# Autodesk Inventor part: 7_68MHZ
Saved by Autodesk Inventor 2016 (Build 200138000, 138)
## iProperties
Created: 2016-04-08
Part Number: 7_68MHZ
Material: Generic
Document SubType Name: Modeling
Designer: Paschalis
Density: 1 g/cm^3
Appearance: HC49U-V, 7_68MHZ
Author: Paschalis
Autodesk Inventor part; units mm, degrees
ref_plane "YZ Plane" through (0, 0, 0) normal (1, 0, 0) x (0, 1, 0)
ref_plane "XZ Plane" through (0, 0, 0) normal (0, 1, 0) x (-1, 0, 0)
ref_plane "XY Plane" through (0, 0, 0) normal (0, 0, 1) x (1, 0, 0)
sketch "HC49U-V, 7_68MHZ_85" plane through (0, 0, 0) normal (0, 0, 1) x (1, 0, 0)
  line L0 (-5.588, 2.794) -> (5.588, 2.794)
  line L1 (5.588, 2.794) -> (5.588, -2.794)
  line L2 (5.588, -2.794) -> (-5.588, -2.794)
  line L3 (-5.588, -2.794) -> (-5.588, 2.794)
  constraints: 8 end point
extrude "Extrusion1" add sketch "HC49U-V, 7_68MHZ_85" along normal blind 1
body "Solid1"
